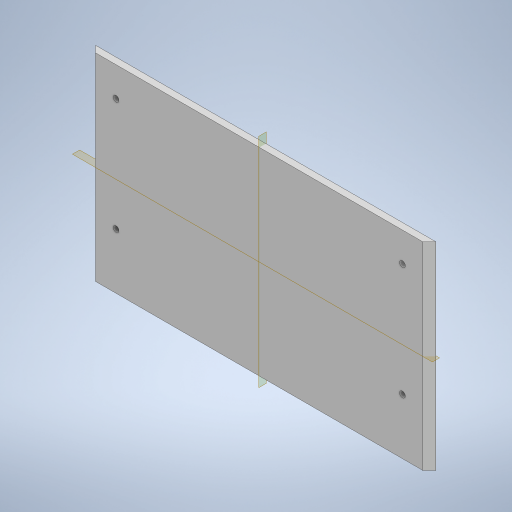
# Autodesk Inventor part: wall-front
Saved by Autodesk Inventor 2023 (Build 270158000, 158)
## iProperties
Created: 2022-10-05
Part Number: wall-front
Material: Generic
Document SubType Name: Modeling
Designer: carso
Density: 1 g/cm^3
Appearance: Default
Author: carso
Autodesk Inventor part; units mm, degrees
ref_plane "YZ Plane" through (0, 0, 0) normal (1, 0, 0) x (0, 1, 0)
ref_plane "XZ Plane" through (0, 0, 0) normal (0, 1, 0) x (-1, 0, 0)
ref_plane "XY Plane" through (0, 0, 0) normal (0, 0, 1) x (1, 0, 0)
sketch "Sketch1" plane through (0, 0, 0) normal (0, 0, 1) x (1, 0, 0)
  line L0 (0, 0) -> (208, 0)
  line L1 (208, 0) -> (208, -121)
  line L2 (208, -121) -> (0, -121)
  line L3 (0, -121) -> (0, 0)
  dimension "d0" = 208
  dimension "d1" = 121
  constraints: 8 end point, 2 parallel, 1 horizontal, 1 perpendicular
  measures "d0" distance of L1.end L2.end
  measures "d1" distance of L0.end L1.end
extrude "Extrusion1" add sketch "Sketch1" along normal blind 4
sketch "Sketch2" plane through (0, 0, 0) normal (0, 0, -1) x (-1, 0, 0)
  line L0 (0, -121) -> (-208, -121) projected
  line L1 (0, -121) -> (-16.5, -121)
  line L2 (-16.5, -121) -> (-16.5, -87)
  line L3 (-16.5, -87) -> (0, -87)
  line L4 (0, -87) -> (0, -121)
  point P0 (0, 0)
  dimension "d4" = 16.5
  dimension "d5" = 34
  constraints: 8 end point, 2 parallel, 1 horizontal, 1 perpendicular
  measures "d4" distance of L2.end L3.end
  measures "d5" distance of L1.end L2.end
hole "Hole1" at (16.5, -87, 0) direction (0, 0, 1) diameter 3.5 depth 8.8
ref_plane "Work Plane1" through (104, -121, 0) normal (-1, 0, 0) x (0, 0, 1)
ref_plane "Work Plane2" through (0, -60.5, 0) normal (0, 1, 0) x (1, 0, 0)
sketch "Sketch3" plane through (0, 0, 4) normal (0, 0, 1) x (1, 0, 0)
  line L0 (208, 0) -> (0, 0) projected
  line L1 (0, 0) -> (16.5, 0)
  line L2 (16.5, 0) -> (16.5, -18)
  line L3 (16.5, -18) -> (0, -18)
  line L4 (0, -18) -> (0, 0)
  dimension "d13" = 16.5
  dimension "d14" = 18
  constraints: 8 end point, 2 parallel, 1 horizontal, 1 perpendicular
  measures "d13" distance of L2.end L3.end
  measures "d14" distance of L1.end L2.end
hole "Hole2" at (16.5, -18, 4) direction (0, 0, -1) diameter 3.5 depth 8.8
mirror "Mirror1" about plane through (104, -121, 0) normal (-1, 0, 0) of "Hole2", "Hole1"
chamfer "Chamfer1" distance 4 angle 45 2 edges at (0, -60.5, 4) (208, -60.5, 4)
body "Solid1"
